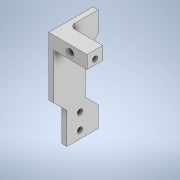
# Autodesk Inventor part: servo-mount
Saved by Autodesk Inventor 2021 (Build 250183000, 183)
## iProperties
Created: 2024-04-27
Part Number: servo-mount
Material: Generic
Document SubType Name: Modeling
Designer: Toby
Density: 1 g/cm^3
Appearance: Default
Author: Toby
Autodesk Inventor part; units mm, degrees
ref_plane "YZ Plane" through (0, 0, 0) normal (1, 0, 0) x (0, 1, 0)
ref_plane "XZ Plane" through (0, 0, 0) normal (0, 1, 0) x (-1, 0, 0)
ref_plane "XY Plane" through (0, 0, 0) normal (0, 0, 1) x (1, 0, 0)
sketch "Sketch1" plane through (0, 0, 0) normal (0, 0, 1) x (1, 0, 0)
  line L0 (-12.5097, 3.9382) -> (-0.5097, 3.9382)
  line L1 (-0.5097, 3.9382) -> (-0.5097, -1.0618)
  line L2 (-0.5097, -1.0618) -> (-12.5097, -1.0618)
  line L3 (-12.5097, -1.0618) -> (-12.5097, 3.9382)
  point P0 (0, 0)
  dimension "d0" = 12
  dimension "d1" = 5
  constraints: 8 end point, 2 parallel, 1 horizontal, 1 perpendicular
  measures "d0" distance of L0.start L0.end
  measures "d1" distance of L0.end L1.end
extrude "Extrusion1" add sketch "Sketch1" along normal blind 6
sketch "Sketch2" plane through (0, 0, 6) normal (0, 0, 1) x (1, 0, 0)
  line L0 (-0.5097, -1.0618) -> (-0.5097, 3.9382) projected
  line L1 (-0.5097, 3.9382) -> (-12.5097, 3.9382) projected
  point P0 (0, 0)
  point P1 (-6.3097, 1.1382)
  dimension "d4" = 5.8
  dimension "d5" = 2.8
  measures "d4" distance from line of L0 point (-6.31, 1.138)
  measures "d5" distance from line of point (-6.31, 1.138) L1
hole "Hole1" at (-6.3097, 1.1382, 6) direction (0, 0, -1) diameter 2 depth 5 tip angle 118 countersink diameter 3 countersink angle 90
sketch "Sketch3" plane through (-0.5097, -1.0618, 0) normal (1, 0, 0) x (0, 0, -1)
  line L0 (0, 5) -> (-6, 5) projected
  line L1 (-6, 0) -> (-6, 5) projected
  point P0 (0, 1.0618)
  point P1 (-3, 2)
  dimension "d13" = 3
  dimension "d14" = 3
  measures "d13" distance from line of point (-3, 2) L0
  measures "d14" distance from line of L1 point (-3, 2)
hole "Hole2" at (-0.5097, 0.9382, 3) direction (-1, 0, 0) diameter 2 depth 3 tip angle 118
sketch "Sketch4" plane through (-12.5097, -1.0618, 0) normal (-1, 0, 0) x (0, 0, 1)
  line L0 (6, 0) -> (6, 5) projected
  line L1 (6, 5) -> (-11, 5)
  line L2 (-11, 5) -> (-11, -34.6)
  line L3 (-11, -34.6) -> (6, -34.6)
  line L4 (6, -34.6) -> (6, 5)
  point P0 (0, 1.0618)
  dimension "d22" = 17
  dimension "d23" = 39.6
  constraints: 8 end point, 2 parallel, 1 horizontal, 1 perpendicular
  measures "d22" distance of L0.end L1.end
  measures "d23" distance of L1.end L2.end
extrude "Extrusion2" add sketch "Sketch4" along normal blind 2
sketch "Sketch5" plane through (-14.5097, -1.0618, 0) normal (-1, 0, 0) x (0, 0, 1)
  line L0 (-11, -34.6) -> (6, -34.6) projected
  line L1 (6, -34.6) -> (6, 5) projected
  point P0 (0, 1.0618)
  point P1 (-4, -25.6)
  point P2 (-4, -31.6)
  dimension "d26" = 3
  dimension "d27" = 9
  dimension "d28" = 10
  dimension "d29" = 10
  measures "d26" distance from line of L0 point (-4, -31.6)
  measures "d27" distance from line of L0 point (-4, -25.6)
  measures "d28" distance from line of L1 point (-4, -25.6)
  measures "d29" distance from line of L1 point (-4, -31.6)
hole "Hole3" at (-14.5097, -26.6618, -4) at (-14.5097, -32.6618, -4) direction (1, 0, 0) diameter 2 depth 3 tip angle 118 countersink diameter 4 countersink angle 90
sketch "Sketch6" plane through (-0.5097, -1.0618, 0) normal (1, 0, 0) x (0, 0, -1)
  line L0 (-6, 5) -> (11, 5) projected
  line L1 (0, 5) -> (0, 0) projected
  line L2 (-6, 5) -> (0, 5)
  line L3 (0, 5) -> (0, 0)
  line L4 (0, 0) -> (-6, 0)
  line L5 (-6, 0) -> (-6, 5)
  circle A0 centre (-3, 2) radius 1 projected
  circle A1 centre (-3, 2) radius 1
  point P0 (0, 1.0618)
  dimension "d37" = 2
  constraints: 8 end point, 2 parallel, 1 centre point, 1 coincident, 1 horizontal, 1 perpendicular
  measures "d37" diameter of A0
extrude "Extrusion3" add sketch "Sketch6" along normal blind 0.8
sketch "Sketch7" plane through (-14.5097, -35.6618, 6) normal (-1, 0, 0) x (0, 0, 1)
  line L0 (-17, 39.6) -> (-17, 0) projected
  line L1 (-17, 31.6) -> (-12, 31.6)
  line L2 (-12, 31.6) -> (-12, 8)
  line L3 (-12, 8) -> (-17, 8)
  line L4 (-17, 8) -> (-17, 31.6)
  line L5 (0, 39.6) -> (-17, 39.6) projected
  line L6 (-17, 0) -> (0, 0) projected
  point P0 (-6, 35.6618)
  point P1 (-10, 0)
  point P2 (-17, 8)
  dimension "d40" = 5
  dimension "d41" = 8
  dimension "d42" = 8
  constraints: 8 end point, 2 parallel, 1 horizontal, 1 perpendicular, 1 point on line
  measures "d40" distance between parallel lines of L0 L2
  measures "d41" distance between parallel lines of L1 L5
  measures "d42" distance between parallel lines of L6 L3
extrude "Extrusion4" cut sketch "Sketch7" against normal blind 2
chamfer "Chamfer1" distance 5 angle 45 2 edges at (-13.5097, -4.0618, -6) (-13.5097, -27.6618, -6)
fillet "Fillet1" radius 2 1 edges at (-12.5097, 1.4382, 0)
sketch "Sketch8" plane through (-14.5097, -35.6618, 6) normal (-1, 0, 0) x (0, 0, 1)
  line L0 (0, 0) -> (0, 39.6) projected
  line L1 (-17, 0) -> (0, 0) projected
  line L2 (0, 12) -> (-5, 12)
  line L3 (-5, 12) -> (-5, 0)
  line L4 (-5, 0) -> (0, 0)
  line L5 (0, 0) -> (0, 12)
  point P0 (-6, 35.6618)
  point P1 (-10, 0)
  dimension "d49" = 5
  dimension "d50" = 12
  constraints: 8 end point, 2 parallel, 2 point on line, 1 horizontal, 1 perpendicular
  measures "d49" distance between parallel lines of L0 L3
  measures "d50" distance between parallel lines of L1 L2
extrude "Extrusion5" cut sketch "Sketch8" against normal blind 10
chamfer "Chamfer2" distance 5 angle 45 1 edges at (-13.5097, -23.6618, 6)
body "Solid1"
